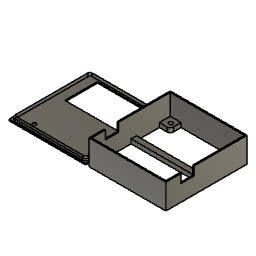
Gehäuse 300 Pushbutton (Autodesk Fusion 360 design; units mm, degrees)
Autodesk Fusion 360 part; units mm, degrees
box "Grundkörper Quader1" add length 73 width 69 height 20 placed x (0, 1, 0) y (-1, 0, 0) z (0, 0, 1) at (69, 0, 0) makes body 1
extrude "Extrusion27" add 1 faces at (69, 48.6667, 6.6667) along direction (1, 0, 0) blind 1.8 on bodies 1 bodies 1
extrude "Extrusion28" add 1 faces at (47.2, 0, 6.6667) along direction (0, -1, 0) blind 1.8 on bodies 1 bodies 1
shell "Schale1" thickness 1.2 removed faces 1 at (23, 24.3333, 20) on bodies 1
extrude "Extrusion1" cut 1 faces at (46.8, 23.5333, 1.2) along direction (0, 0, -1) blind 1.2 on bodies 1 bodies 1
box "Grundkörper Quader7" add length 10 width 10 height 4 placed x (0, 1, 0) y (-1, 0, 0) z (0, 0, 1) at (11.6701, 1.5796, 0) separate body makes body 2
move_body "Verschieben58" bodies 2 to x (1, 0, 0) y (0, 1, 0) z (0, 0, 1) at (0, -2.1796, 0)
cylinder "Grundkörper Zylinder2" cut diameter 3.5 height -4 placed x (1, 0, 0) y (0, 1, 0) z (0, 0, 1) at (6.2481, 6.6899, 4) bodies 2
move_face "Fläche verschieben12" to x (1, 0, 0) y (0, 1, 0) z (0, 0, 1) at (1, 0, 0) 1 faces at (7.9894, 6.5157, 2.6667) on bodies 2
move_face "Fläche verschieben5" to x (1, 0, 0) y (0, 1, 0) z (0, 0, 1) at (0, -1.5, 0) 1 faces at (8.9894, 6.5157, 2.6667) on bodies 2
move_face "Fläche verschieben7" to x (1, 0, 0) y (0, 1, 0) z (0, 0, 1) at (0, -0.25, 0) 1 faces at (8.9894, 5.0157, 2.6667) on bodies 2
move_face "Fläche verschieben6" to x (1, 0, 0) y (0, 1, 0) z (0, 0, 1) at (-0.25, 0, 0) 1 faces at (8.9894, 4.7657, 2.6667) on bodies 2
move_face "Fläche verschieben13" to x (1, 0, 0) y (0, 1, 0) z (0, 0, 1) at (1, 0, 0) 1 faces at (8.7394, 4.7657, 2.6667) on bodies 2
move_face "Fläche verschieben8" to x (1, 0, 0) y (0, 1, 0) z (0, 0, 1) at (0, 1.2, 0) 1 faces at (9.7394, 4.7657, 2.6667) on bodies 2
move_face "Fläche verschieben14" to x (1, 0, 0) y (0, 1, 0) z (0, 0, 1) at (0, -0.5, 0) 1 faces at (9.7394, 5.9657, 2.6667) on bodies 2
copy_body "Körper kopieren/einfügen3" bodies 2 makes body 3
move_body "Verschieben34" bodies 3 to x (1, 0, 0) y (0, 1, 0) z (0, 0, 1) at (0, 60, 0)
copy_body "Körper kopieren/einfügen4" bodies 2 makes body 4
move_face "Fläche verschieben11" to x (1, 0, 0) y (0, 1, 0) z (0, 0, 1) at (1, -1.5, 0) 1 faces at (9.6107, 66.3197, 1.3333) on bodies 3
move_face "Fläche verschieben9" to x (1, 0, 0) y (0, 1, 0) z (0, 0, 1) at (0, -2.4, 0) 1 faces at (10.6107, 64.8197, 1.3333) on bodies 3
move_body "Verschieben59" bodies 3 to x (1, 0, 0) y (0, 1, 0) z (0, 0, 1) at (0, 2.4, 0)
move_body "Verschieben60" bodies 3 to x (1, 0, 0) y (0, 1, 0) z (0, 0, 1) at (-0.4701, 0, 0)
move_body "Verschieben61" bodies 4 to x (1, 0, 0) y (0, 1, 0) z (0, 0, 1) at (-0.4701, 0, 0)
move_body "Verschieben62" bodies 4 to x (1, 0, 0) y (0, 1, 0) z (0, 0, 1) at (60, 0, 0)
move_body "Verschieben63" bodies 4 to x (1, 0, 0) y (0, 1, 0) z (0, 0, 1) at (-10, 0, 0)
move_body "Verschieben64" bodies 4 to x (1, 0, 0) y (0, 1, 0) z (0, 0, 1) at (8.4, 0, 0)
move_body "Verschieben65" bodies 2 to x (1, 0, 0) y (0, 1, 0) z (0, 0, 1) at (-0.4701, 0, 0)
copy_body "Körper kopieren/einfügen7" bodies 4 makes body 5
move_body "Verschieben68" bodies 5 to x (1, 0, 0) y (0, 1, 0) z (0, 0, 1) at (0, 40, 0)
move_face "Fläche verschieben10" to x (1, 0, 0) y (0, 1, 0) z (0, 0, 1) at (0, -2.4, 0) 1 faces at (67.5406, 44.9602, 2.6667) on bodies 5
move_face "Fläche verschieben15" to x (1, 0, 0) y (0, 1, 0) z (0, 0, 1) at (0.5, -0.5, 0) 1 faces at (67.5406, 42.5602, 2.6667) on bodies 5
move_body "Verschieben69" bodies 5 to x (1, 0, 0) y (0, 1, 0) z (0, 0, 1) at (0, 22.4, 0)
fillet "Abrundung14" radius 3 2 edges at (59.6, 9.4, 2) (59.6, 61.8, 2) on bodies 4 5
fillet "Abrundung15" radius 3 2 edges at (11.2, 9.4, 2) (11.2, 61.8, 2) on bodies 2 3
move_face "Fläche verschieben16" to x (1, 0, 0) y (0, 1, 0) z (0, 0, 1) at (0.5, -1, 0) 1 faces at (64.77, 6.952, 2.6667) on bodies 4
move_face "Fläche verschieben17" to x (1, 0, 0) y (0, 1, 0) z (0, 0, 1) at (-1.5, 2.5, 0) 1 faces at (6.8835, 64.7385, 1.3333) on bodies 3
move_face "Fläche verschieben18" to x (1, 0, 0) y (0, 1, 0) z (0, 0, 1) at (-2, 0, 0) 1 faces at (67.823, 66.1966, 2.6667) on bodies 5
move_face "Fläche verschieben19" to x (1, 0, 0) y (0, 1, 0) z (0, 0, 1) at (-2, 0, 0) 1 faces at (65.27, 5.952, 2.6667) on bodies 4
move_face "Fläche verschieben20" to x (1, 0, 0) y (0, 1, 0) z (0, 0, 1) at (0, 0.3, 0) 1 faces at (66.1693, 4.4657, 2.6667) on bodies 4
move_face "Fläche verschieben21" to x (1, 0, 0) y (0, 1, 0) z (0, 0, 1) at (-0.6, 0, 0) 1 faces at (9.2693, 5.4657, 2.6667) on bodies 2
move_face "Fläche verschieben22" to x (1, 0, 0) y (0, 1, 0) z (0, 0, 1) at (0, -0.7, 0) 1 faces at (8.6693, 5.4657, 2.6667) on bodies 2
box "Grundkörper Quader16" add length 5 width 68.4 height -4 placed x (0, -1, 0) y (-1, 0, 0) z (0, 0, -1) at (69.6, 39.1587, 0) separate body makes body 6
move_body "Verschieben74" bodies 6 to x (1, 0, 0) y (0, 1, 0) z (0, 0, 1) at (0, 1.6, 0)
box "Grundkörper Quader22" add length 74.8 width 70.8 height 1.2 placed x (0, 1, 0) y (-1, 0, 0) z (0, 0, 1) at (70.8, -1.8, 20) separate body makes body 7
box "Grundkörper Quader23" add length 72.3 width 68.3 height -3 placed x (0, 1, 0) y (-1, 0, 0) z (0, 0, 1) at (69.5, -0.6, 20) separate body makes body 8
move_body "Verschieben89" bodies 8 to x (1, 0, 0) y (0, 1, 0) z (0, 0, 1) at (0.05, -0.05, 0)
fillet "Abrundung18" radius 3 3 edges at (69.55, -0.65, 18.5) (69.55, 71.65, 18.5) (1.25, -0.65, 18.5) on bodies 8
fillet "Abrundung19" radius 3 1 edges at (1.25, 71.65, 18.5) on bodies 8
shell "Schale5" thickness 1.2 removed faces 1 at (46.7833, 24.45, 20) on bodies 8
extrude "Extrusion46" cut 1 faces at (46.3833, 46.55, 18.2) along direction (0, 0, -1) blind 1.2 on bodies 8 bodies 8
chamfer "Fase6" distance 1.2 angle 45 8 edges at (35.4, -0.65, 17) (2.1287, 0.2287, 17) (1.25, 35.5, 17) (2.1287, 70.7713, 17) (35.4, 71.65, 17) (68.6713, 70.7713, 17) (69.55, 35.5, 17) (68.6713, 0.2287, 17) on bodies 8
box "Grundkörper Quader24" add length 30 width 47 height -20 placed x (0, 1, 0) y (-1, 0, 0) z (0, 0, 1) at (56, 40, 21.2) separate body makes body 9
move_body "Verschieben90" bodies 9 to x (1, 0, 0) y (0, 1, 0) z (0, 0, 1) at (4, -1, 0)
combine "Kombinieren11" operation cut target body 7 tool bodies 9
move_body "Verschieben91" bodies 7 8 to x (-1, 0, 0) y (0, 1, 0) z (0, 0, -1) at (-3, 0, 21)
box "Grundkörper Quader25" add length 12 width 81.567 height -5 placed x (0, 1, 0) y (-1, 0, 0) z (0, 0, 1) at (81.5675, 12.1425, 20) separate body makes body 10
move_body "Verschieben92" bodies 10 to x (1, 0, 0) y (0, 1, 0) z (0, 0, 1) at (-3, 0, 0)
combine "Kombinieren12" operation cut target body 1 tool bodies 10
cylinder "Grundkörper Zylinder5" add diameter 3 height -5 placed x (1, 0, 0) y (0, 1, 0) z (0, 0, 1) at (-14.2242, 6.6053, 1) separate body makes body 11
move_body "Verschieben93" bodies 11 to x (1, 0, 0) y (0, 1, 0) z (0, 0, 1) at (0, -0.4, 0)
move_body "Verschieben94" bodies 11 to x (1, 0, 0) y (0, 1, 0) z (0, 0, 1) at (-5, 0, 0)
move_body "Verschieben95" bodies 11 to x (1, 0, 0) y (0, 1, 0) z (0, 0, 1) at (-39, 0, 0)
combine "Kombinieren13" operation cut target body 7 tool bodies 11
chamfer "Fase7" distance 1 angle 45 1 edges at (-57.6818, 4.8068, -0.2) on bodies 7
extrude "Extrusion47" add 1 faces at (24, -1.4, 20) along direction (0, 0, 1) blind 3 on bodies 1 bodies 1
extrude "Extrusion48" add 1 faces at (46.8, 72.6, 20) along direction (0, 0, 1) blind 3 on bodies 1 bodies 1
extrude "Extrusion36" [suppressed]
extrude "Extrusion37" [suppressed]
extrude "Extrusion38" [suppressed]
extrude "Extrusion39" [suppressed]
extrude "Extrusion40" [suppressed]
extrude "Extrusion41" [suppressed]
extrude "Extrusion42" [suppressed]
extrude "Extrusion44" [suppressed]
extrude "Extrusion45" [suppressed]
named bodies: "Rahmen", "Auflage 1", "Auflage 2", "Auflage 3", "Auflage 4", "Strebe", "Deckel", "Deckelrahmen"
